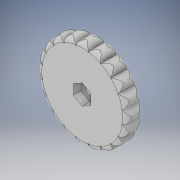
# Autodesk Inventor part: 20_gear
Saved by Autodesk Inventor 2019 (Build 230136000, 136)
## iProperties
Created: 2020-06-16
Part Number: 20_gear
Material: Generic
Document SubType Name: Modeling
Designer: UC2
Density: 1 g/cm^3
Appearance: Default
Author: UC2
Autodesk Inventor part; units mm, degrees
ref_plane "YZ Plane" through (0, 0, 0) normal (1, 0, 0) x (0, 1, 0)
ref_plane "XZ Plane" through (0, 0, 0) normal (0, 1, 0) x (-1, 0, 0)
ref_plane "XY Plane" through (0, 0, 0) normal (0, 0, 1) x (1, 0, 0)
sketch "Skizze1" plane through (0, 0, 0) normal (0, 0, 1) x (1, 0, 0)
  line L0 (-20.3, 0) -> (20.3, 0) construction
  line L1 (0, -20.3) -> (0, 20.3) construction
  circle A0 centre (0, 0) radius 12.5
  circle A1 centre (0, 0) radius 1.6
  arc A2 (1.99359, 12.34) -> (-1.99359, 12.34) centre (0, 12.5) ccw
  circle A3 centre (0, 0) radius 14.5 construction
  dimension "d1" = 3.2
  dimension "d2" = 2
  dimension "d3" = 29
  constraints: 5 point on circle, 4 centre point, 3 coincident, 1 point on line, 1 tangent
  measures "d1" diameter of A1
  measures "d2" radius of A2
  measures "d3" diameter of A3
extrude "Extrusion1" add sketch "Skizze1" along normal blind 5
pattern_circular "Runde Anordnung1" count 20 over 360 about axis through (0, 0, -10) along (0, 0, 1) of "Extrusion1"
sketch "Skizze2" plane through (0, 0, 5) normal (0, 0, 1) x (1, 0, 0)
  circle A0 centre (0, 0) radius 1.6 construction
  arc A1 (-1.997038, 12.608803) -> (-5.795631, 11.374566) centre (-3.862712, 11.888206) ccw construction
  arc A2 (-5.795631, 11.374566) -> (-9.026907, 9.026907) centre (-7.347316, 10.112712) ccw construction
  arc A3 (-9.026907, 9.026907) -> (-11.374566, 5.795631) centre (-10.112712, 7.347316) ccw construction
  arc A4 (-11.374566, 5.795631) -> (-12.608803, 1.997038) centre (-11.888206, 3.862712) ccw construction
  arc A5 (-12.608803, 1.997038) -> (-12.608803, -1.997038) centre (-12.5, 0) ccw construction
  arc A6 (-12.608803, -1.997038) -> (-11.374566, -5.795631) centre (-11.888206, -3.862712) ccw construction
  arc A7 (-11.374566, -5.795631) -> (-9.026907, -9.026907) centre (-10.112712, -7.347316) ccw construction
  arc A8 (-9.026907, -9.026907) -> (-5.795631, -11.374566) centre (-7.347316, -10.112712) ccw construction
  arc A9 (-5.795631, -11.374566) -> (-1.997038, -12.608803) centre (-3.862712, -11.888206) ccw construction
  arc A10 (-1.997038, -12.608803) -> (1.997038, -12.608803) centre (0, -12.5) ccw construction
  arc A11 (1.997038, -12.608803) -> (5.795631, -11.374566) centre (3.862712, -11.888206) ccw construction
  arc A12 (5.795631, -11.374566) -> (9.026907, -9.026907) centre (7.347316, -10.112712) ccw construction
  arc A13 (9.026907, -9.026907) -> (11.374566, -5.795631) centre (10.112712, -7.347316) ccw construction
  arc A14 (11.374566, -5.795631) -> (12.608803, -1.997038) centre (11.888206, -3.862712) ccw construction
  arc A15 (12.608803, -1.997038) -> (12.608803, 1.997038) centre (12.5, 0) ccw construction
  arc A16 (12.608803, 1.997038) -> (11.374566, 5.795631) centre (11.888206, 3.862712) ccw construction
  arc A17 (11.374566, 5.795631) -> (9.026907, 9.026907) centre (10.112712, 7.347316) ccw construction
  arc A18 (9.026907, 9.026907) -> (5.795631, 11.374566) centre (7.347316, 10.112712) ccw construction
  arc A19 (5.795631, 11.374566) -> (1.997038, 12.608803) centre (3.862712, 11.888206) ccw construction
  arc A20 (1.997038, 12.608803) -> (-1.997038, 12.608803) centre (0, 12.5) ccw construction
  line L0 (-20.3, 0) -> (20.3, 0) construction
  line L1 (0, -20.3) -> (0, 20.3) construction
  line L2 (0, 3.25) -> (2.814583, 1.625)
  line L3 (2.814583, 1.625) -> (2.814583, -1.625)
  line L4 (2.814583, -1.625) -> (0, -3.25)
  line L5 (0, -3.25) -> (-2.814583, -1.625)
  line L6 (-2.814583, -1.625) -> (-2.814583, 1.625)
  line L7 (-2.814583, 1.625) -> (0, 3.25)
  dimension "d9" = 6.5
  constraints: 12 end point, 1 coincident, 1 point on line, 13 other
  measures "d9" distance of L4.end L2.start
extrude "Extrusion2" cut sketch "Skizze2" against normal blind 2.5
sketch "Sketch3" plane through (0, 0, 0) normal (1, 0, 0) x (0, 1, 0)
  line L0 (1.625, 5) -> (3.25, 5) construction
  line L1 (3.25, 5) -> (1.625, 5) construction
  line L2 (1.625, 5) -> (-1.625, 5) construction
  line L3 (-1.625, 5) -> (-3.25, 5) construction
  line L4 (-3.25, 5) -> (-1.625, 5) construction
  line L5 (-1.625, 5) -> (1.625, 5) construction
  line L6 (12.608803, 5) -> (11.374566, 5) construction
  line L7 (11.374566, 5) -> (9.026907, 5) construction
  line L8 (9.026907, 5) -> (5.795631, 5) construction
  line L9 (5.795631, 5) -> (1.997038, 5) construction
  line L10 (1.997038, 5) -> (-1.997038, 5) construction
  line L11 (-1.997038, 5) -> (-5.795631, 5) construction
  line L12 (-5.795631, 5) -> (-9.026907, 5) construction
  line L13 (-9.026907, 5) -> (-11.374566, 5) construction
  line L14 (-11.374566, 5) -> (-12.608803, 5) construction
  line L15 (-12.608803, 5) -> (-12.608803, 5) construction
  line L16 (-12.608803, 5) -> (-11.374566, 5) construction
  line L17 (-11.374566, 5) -> (-9.026907, 5) construction
  line L18 (-9.026907, 5) -> (-5.795631, 5) construction
  line L19 (-5.795631, 5) -> (-1.997038, 5) construction
  line L20 (-1.997038, 5) -> (1.997038, 5) construction
  line L21 (1.997038, 5) -> (5.795631, 5) construction
  line L22 (5.795631, 5) -> (9.026907, 5) construction
  line L23 (9.026907, 5) -> (11.374566, 5) construction
  line L24 (11.374566, 5) -> (12.608803, 5) construction
  line L25 (12.608803, 5) -> (12.608803, 5) construction
  line L26 (12.608803, 0) -> (12.608803, 0) construction
  line L27 (11.374566, 0) -> (12.608803, 0) construction
  line L28 (9.026907, 0) -> (11.374566, 0) construction
  line L29 (5.795631, 0) -> (9.026907, 0) construction
  line L30 (1.997038, 0) -> (5.795631, 0) construction
  line L31 (-1.997038, 0) -> (1.997038, 0) construction
  line L32 (-5.795631, 0) -> (-1.997038, 0) construction
  line L33 (-9.026907, 0) -> (-5.795631, 0) construction
  line L34 (-11.374566, 0) -> (-9.026907, 0) construction
  line L35 (-12.608803, 0) -> (-11.374566, 0) construction
  line L36 (-12.608803, 0) -> (-12.608803, 0) construction
  line L37 (-11.374566, 0) -> (-12.608803, 0) construction
  line L38 (-9.026907, 0) -> (-11.374566, 0) construction
  line L39 (-5.795631, 0) -> (-9.026907, 0) construction
  line L40 (-1.997038, 0) -> (-5.795631, 0) construction
  line L41 (1.997038, 0) -> (-1.997038, 0) construction
  line L42 (5.795631, 0) -> (1.997038, 0) construction
  line L43 (9.026907, 0) -> (5.795631, 0) construction
  line L44 (11.374566, 0) -> (9.026907, 0) construction
  line L45 (12.608803, 0) -> (11.374566, 0) construction
  line L46 (1.6, 0) -> (-1.6, 0) construction
  line L47 (12.608803, 0) -> (12.608803, 5) construction
  line L48 (12.608803, 5) -> (12.608803, 5) construction
  line L49 (12.608803, 5) -> (12.608803, 0) construction
  line L50 (12.608803, 0) -> (12.608803, 0) construction
  line L51 (-12.608803, 0) -> (-12.608803, 5) construction
  line L52 (-12.608803, 5) -> (-12.608803, 5) construction
  line L53 (-12.608803, 0) -> (-12.608803, 5) construction
  line L54 (-12.608803, 0) -> (-12.608803, 0) construction
  line L55 (-14.5, 0) -> (-14.5, 5) construction
  line L56 (-12.608803, 5) -> (-14.5, 5) construction
  line L57 (-12.608803, 0) -> (-14.5, 0) construction
  line L58 (0, -1) -> (0, 6)
  line L59 (14.5, 0) -> (14.5, 5) construction
  line L60 (14.5, 5) -> (12.608803, 5) construction
  line L61 (14.5, 0) -> (12.608803, 0) construction
  line L62 (13, 5) -> (14.5, 5)
  line L63 (14.5, 5) -> (14.5, 3.5)
  line L64 (12.608803, 0) -> (12.608803, 5) construction
  line L65 (12.608803, 2.5) -> (14.5, 2.5) construction
  arc A0 (14.5, 3.5) -> (13, 5) centre (13, 3.5) ccw
  line L66 (13, 0) -> (14.5, 0)
  arc A1 (13, 0) -> (14.5, 1.5) centre (13, 1.5) ccw
  line L67 (14.5, 1.5) -> (14.5, 0)
  point P0 (0, 0)
  dimension "d13" = 1.5
  dimension "d14" = 1.5
  dimension "d15" = 1.5
  constraints: 10 end point, 4 point on circle, 3 symmetric about line, 2 centre point, 2 point on line, 1 collinear, 1 midpoint, 1 vertical, 3 other
  measures "d13" radius of A0
  measures "d14" distance of L59.end L62.start
  measures "d15" distance of L59.end L63.end
revolve "Revolution1" cut sketch "Sketch3" angle 360 about axis through (0, 0, -10) along (0, 0, 1)
